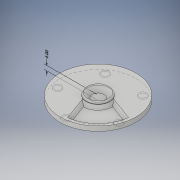
# Autodesk Inventor part: dissection_platform_v01
Saved by Autodesk Inventor 2019 (Build 230136000, 136)
## iProperties
Created: 2018-12-14
Part Number: dissection_platform_v01
Material: Generic
Document SubType Name: Modeling
Designer: Wilson Lab
Density: 1 g/cm^3
Appearance: Default
Author: Wilson Lab
Autodesk Inventor part; units mm, degrees
ref_plane "YZ Plane" through (0, 0, 0) normal (1, 0, 0) x (0, 1, 0)
ref_plane "XZ Plane" through (0, 0, 0) normal (0, 1, 0) x (-1, 0, 0)
ref_plane "XY Plane" through (0, 0, 0) normal (0, 0, 1) x (1, 0, 0)
sketch "Base Material Sketch" plane through (0, 0, 0) normal (0, 1, 0) x (-1, 0, 0)
  circle A0 centre (0, 0) radius 32.5
  dimension "d0" = 65
  constraints: 1 centre point, 1 coincident
  measures "d0" diameter of A0
extrude "Base Material Extrusion" add sketch "Base Material Sketch" along normal blind 4
sketch "Magnet Recess" plane through (0, 0, 0) normal (0, -1, 0) x (1, 0, 0)
  circle A0 centre (0, 0) radius 32.5 projected
  circle A1 centre (0, 27.5) radius 3.25
  line L0 (0, 0) -> (0, 32.5) construction
  circle A2 centre (0, 0) radius 32.5 construction
  circle A3 centre (-26.1541, 8.498) radius 3.25
  circle A4 centre (-16.1641, -22.248) radius 3.25
  circle A5 centre (16.1641, -22.248) radius 3.25
  circle A6 centre (26.1541, 8.498) radius 3.25
  dimension "d3" = 6.5
  dimension "d4" = 5
  dimension "d7" = 360
  constraints: 5 centre point, 2 end point, 1 point on line, 1 vertical, 1 vertical alignment, 12 other
  measures "d3" diameter of A1
  measures "d4" distance of A1.centre L0.end
extrude "Bottom Magnet Recess" cut sketch "Magnet Recess" against normal blind 1 contours A1 | A3 | A4 | A5 | A6
sketch "Central Well" plane through (0, 4, 0) normal (0, 1, 0) x (1, 0, 0)
  circle A0 centre (0, 0) radius 32.5 construction
  circle A1 centre (0, 0) radius 5
  dimension "d12" = 10
  constraints: 1 centre point, 1 coincident
  measures "d12" diameter of A1
extrude "Well Recess" cut sketch "Central Well" against normal blind 2
sketch "Sketch6" plane through (0, 4, 0) normal (0, 1, 0) x (1, 0, 0)
  circle A0 centre (0, 0) radius 9
  circle A1 centre (0, 0) radius 10
  dimension "d22" = 18
  dimension "d23" = 20
  constraints: 2 centre point, 2 coincident
  measures "d22" diameter of A0
  measures "d23" diameter of A1
extrude "Well Wall" add sketch "Sketch6" along normal blind 2
sketch "kimwipe recess sketch" plane through (0, 4, 0) normal (0, 1, 0) x (1, 0, 0)
  circle A0 centre (0, 0) radius 32.5 construction
  circle A1 centre (0, 0) radius 10 construction
  circle A2 centre (0, 0) radius 5 construction
  arc A3 (0, -12.5) -> (12.5, 0) centre (0, 0) ccw
  circle A4 centre (0, 0) radius 32.5 construction
  line L0 (0, 0) -> (-27.5, 0) construction
  line L1 (0, 0) -> (27.5, 0) construction
  line L2 (0, 0) -> (0, -27.5) construction
  line L3 (12.5, 0) -> (26.9896, -5.2738)
  line L4 (0, -12.5) -> (5.2738, -26.9896)
  arc A5 (5.2738, -26.9896) -> (26.9896, -5.2738) centre (0, 0) ccw
  dimension "d31" = 2.5
  dimension "d34" = 20
  dimension "d35" = 20
  dimension "d36" = 27.5
  constraints: 10 end point, 4 point on circle, 3 coincident, 2 centre point, 2 horizontal, 2 point on line, 1 perpendicular
  measures "d31" radial gap between concentric circles of A3 A1
  measures "d34" angle of L1 L3
  measures "d35" angle of L4 L2
  measures "d36" radius of A5
chamfer "Well Chamfer" distance 2 angle 45 2 edges at (-5, 4, 0) (-9, 4, 0)
fillet "Well Wall Fillet" radius 2 1 edges at (-10, 6, 0)
extrude "Extrusion6" cut sketch "kimwipe recess sketch" against normal blind 2.5
chamfer "Chamfer3" distance 2.5 angle 45 4 edges at (2.6369, 4, 19.7448) (8.8388, 4, 8.8388) (19.7448, 4, 2.6369) (19.4454, 4, 19.4454)
body "Solid1"
